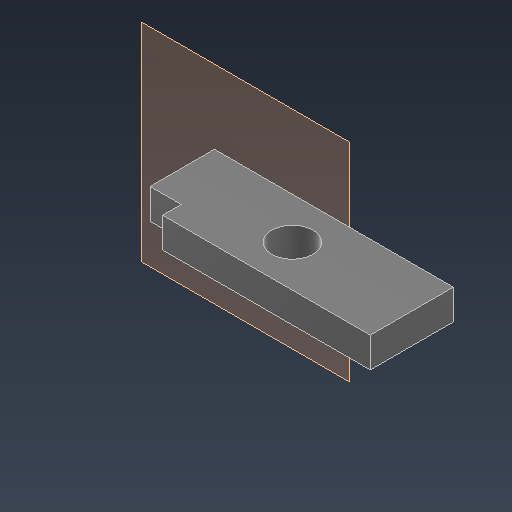
# Autodesk Inventor part: Cap Pulley Support V2 Pt2
Saved by Autodesk Inventor 2021.3 (Build 253353000, 353)
## iProperties
Created: 2022-07-27
Part Number: Cap Pulley Support V2 Pt2
Material: Thermoplastic Resin
Document SubType Name: Modeling
Designer: david
Density: 1.28 g/cm^3
Appearance: Smooth - Black
Author: david
Autodesk Inventor part; units mm, degrees
ref_plane "YZ Plane" through (0, 0, 0) normal (1, 0, 0) x (0, 1, 0)
ref_plane "XZ Plane" through (0, 0, 0) normal (0, 1, 0) x (-1, 0, 0)
ref_plane "XY Plane" through (0, 0, 0) normal (0, 0, 1) x (1, 0, 0)
ref_plane "Work Plane1" through (0, 0, 5) normal (0, 0, 1) x (1, 0, 0)
sketch "Sketch1" plane through (0, 0, 5) normal (0, 0, 1) x (1, 0, 0)
  line L0 (0, 0) -> (20, 0)
  line L1 (20, 0) -> (20, 2.9)
  line L2 (20, 2.9) -> (0, 2.9)
  line L3 (0, 2.9) -> (0, 0)
  dimension "d2" = 20
  dimension "d1" = 2.9
  constraints: 8 end point, 2 parallel, 1 perpendicular
  measures "d2" distance of L0.end L0.start
  measures "d1" distance of L2.end L0.start
extrude "Extrusion1" add sketch "Sketch1" along normal blind 8
sketch "Sketch2" plane through (0, 0, 5) normal (-1, 0, 0) x (0, 0, 1)
  line L0 (0, 0) -> (0, 2.9) projected
  line L1 (0, 0) -> (8, 0) projected
  line L2 (0, 0) -> (6.2, 0)
  line L3 (6.2, 0) -> (6.2, 2.9)
  line L4 (6.2, 2.9) -> (0, 2.9)
  line L5 (0, 2.9) -> (0, 0)
  point P0 (-13, 0)
  dimension "d6" = 6.2
  constraints: 8 end point, 2 parallel, 1 perpendicular, 1 point on line
  measures "d6" distance between parallel lines of L3 L0
extrude "Extrusion2" add sketch "Sketch2" along normal blind 3
sketch "Sketch3" plane through (20, 2.9, 5) normal (0, 1, 0) x (0, 0, 1)
  line L0 (0, 0) -> (0, -23) projected
  line L1 (8, -20) -> (8, 0) projected
  line L2 (0, -20) -> (8, -20)
  line L3 (4, -20) -> (4, -11.5)
  circle A0 centre (4, -11.5) radius 2
  point P0 (-13, -20)
  dimension "d11" = 8.5
  dimension "d10" = 4
  constraints: 4 end point, 1 centre point, 1 coincident, 1 midpoint, 1 perpendicular, 1 point on line, 1 vertical
  measures "d11" distance of L3.start L3.end
  measures "d10" diameter of A0
extrude "Extrusion3" cut sketch "Sketch3" against normal through all
body "Solid1"
